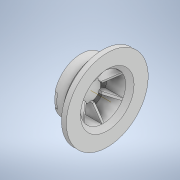
# Autodesk Inventor part: Крышка цилиндра 1
Saved by Autodesk Inventor 2021 (Build 250183000, 183)
## iProperties
Created: 2020-10-25
Part Number: Крышка цилиндра 1
Material: Типовые
Document SubType Name: Modeling
Designer: Тимоха
Density: 1 g/cm^3
Appearance: По умолчанию
Author: Тимоха
Autodesk Inventor part; units mm, degrees
ref_plane "YZ Plane" through (0, 0, 0) normal (1, 0, 0) x (0, 1, 0)
ref_plane "XZ Plane" through (0, 0, 0) normal (0, 1, 0) x (-1, 0, 0)
ref_plane "XY Plane" through (0, 0, 0) normal (0, 0, 1) x (1, 0, 0)
sketch "Эскиз1" plane through (0, 0, 0) normal (0, 0, 1) x (1, 0, 0)
  line L0 (0, 0) -> (0, 190)
  line L1 (0, 190) -> (112, 190)
  line L2 (112, 190) -> (112, 240)
  line L3 (112, 240) -> (152, 240)
  line L4 (152, 240) -> (152, 290)
  line L5 (152, 290) -> (187, 290)
  line L6 (187, 290) -> (187, 190)
  line L7 (0, 190) -> (0, 160)
  line L8 (0, 160) -> (268.4083, 160)
  line L9 (187, 190) -> (218.141, 190) construction
  line L10 (187, 190) -> (157, 160)
  line L11 (0, 160) -> (30, 160)
  line L12 (30, 160) -> (30, 70)
  line L13 (30, 70) -> (70, 70)
  line L14 (70, 70) -> (70, 0)
  line L15 (70, 0) -> (45, 0)
  line L16 (45, 0) -> (45, 45)
  line L17 (45, 45) -> (0, 45)
  line L18 (135.1883, 240) -> (135.1883, 235)
  line L19 (135.1883, 235) -> (140.1883, 235)
  line L20 (140.1883, 235) -> (140.1883, 240)
  dimension "d0" = 190
  dimension "d1" = 112
  dimension "d2" = 50
  dimension "d3" = 40
  dimension "d4" = 50
  dimension "d5" = 35
  dimension "d6" = 100
  dimension "d9" = 30
  dimension "d12" = 45
  dimension "d13" = 30
  dimension "d14" = 90
  dimension "d15" = 40
  dimension "d16" = 25
  dimension "d17" = 45
  dimension "d35" = 5
  dimension "d36" = 5
  constraints: 42 end point, 13 perpendicular, 6 point on line, 3 vertical, 2 horizontal
  measures "d0" distance of L0.start L0.end
  measures "d1" distance of L0.end L1.end
  measures "d2" distance of L1.end L2.end
  measures "d3" distance of L2.end L3.end
  measures "d4" distance of L3.end L4.end
  measures "d5" distance of L4.end L5.end
  measures "d6" distance of L5.end L6.end
  measures "d9" distance of L0.end L7.end
  measures "d12" angle of L8 L10
  measures "d13" distance of L7.end L11.end
  measures "d14" distance of L11.end L12.end
  measures "d15" distance of L12.end L13.end
  measures "d16" distance of L14.end L15.end
  measures "d17" distance of L15.end L16.end
  measures "d35" distance of L18.start L18.end
  measures "d36" distance of L18.end L19.end
revolve "Вращение1" add sketch "Эскиз1" angle 360 about axis through (70, 0, 0) along (-1, 0, 0) contours L0 L8 L12 L13 L14 L15 L16 L17 | L0 L1 L2 L3 L18 L19 L20 L4 L5 L6 L10 L8
sketch "Эскиз2" plane through (0, 0, 0) normal (0, 0, 1) x (1, 0, 0)
  line L0 (30, -160) -> (30, 160) projected
  line L1 (30, 70) -> (70, 70) projected
  line L2 (157, 160) -> (30, 160) projected
  line L3 (30, -70) -> (30, 70) projected
  line L4 (30, 70) -> (30, 65)
  line L5 (30, 65) -> (90, 65)
  line L6 (90, 65) -> (157, 160)
  point P0 (0, 0)
  dimension "d25" = 5
  dimension "d26" = 60
  constraints: 6 end point, 1 parallel, 1 point on line
  measures "d25" distance of L1.start L4.end
  measures "d26" distance of L4.end L5.end
extrude "Выдавливание1" add sketch "Эскиз2" along normal mid plane 15
pattern_circular "Круговой массив1" count 6 over 360 about axis through (169.5, 0, 0) along (1, 0, 0) of "Выдавливание1"
sketch "Эскиз6" plane through (0, 0, 0) normal (0, 1, 0) x (-1, 0, 0)
  line L0 (0, -190) -> (-112, -190) projected
  line L1 (0, 190) -> (0, -190) projected
  line L2 (0, -190) -> (0, -186)
  line L3 (0, -186) -> (-19, -186)
  line L4 (-19, -186) -> (-19, -190)
  line L5 (0, -186) -> (-19, -190)
  line L6 (37.4, 0) -> (-224.4, 0) projected
  point P0 (0, 0)
  dimension "d37" = 4
  dimension "d38" = 19
  constraints: 8 end point, 2 perpendicular, 2 point on line
  measures "d37" distance of L0.start L2.end
  measures "d38" distance of L2.end L3.end
revolve "Вращение2" cut sketch "Эскиз6" angle 30 mid plane about axis through (169.5, 0, 0) along (1, 0, 0) contours L0 L5 L1
pattern_circular "Круговой массив2" count 2 over 360 about axis through (169.5, 0, 0) along (1, 0, 0) of "Вращение2"
